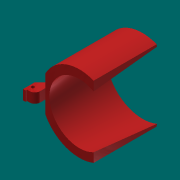
# Autodesk Inventor part: 知能ロボコン吸引部２.1.2
Saved by Autodesk Inventor 2013 (Build 170138000, 138)
## iProperties
Created: 2014-11-21
Part Number: 知能ロボコン吸引部２.1.2
Material: 一般
Document SubType Name: Modeling
Designer: horumo136
Density: 1 g/cm^3
Author: horumo136
Autodesk Inventor part; units mm, degrees
sketch "スケッチ1" plane through (0, 0, 0) normal (0, 0, 1) x (1, 0, 0)
  line L0 (0, 0) -> (32, 0)
  line L1 (0, 0) -> (0, 30)
  line L2 (0, 30) -> (35, 30)
  line L3 (35, 30) -> (32, 0)
  line L4 (32, 0) -> (33.9901, -0.199)
  line L5 (33.9901, -0.199) -> (36.9901, 29.801)
  line L6 (36.9901, 29.801) -> (35, 30)
  line L7 (0, 0) -> (0, -80)
  line L8 (0, -80) -> (26.01, -80)
  line L9 (32, 0) -> (24.0199, -79.801)
  line L10 (33.9901, -0.199) -> (26.01, -80)
  line L11 (26.01, -80) -> (24.0199, -79.801)
  line L12 (26.01, -80) -> (36.9901, -80)
  line L13 (36.9901, -80) -> (36.9901, 29.801)
  line L14 (24.0199, -79.801) -> (24, -80)
  dimension "d0" = 32
  dimension "d1" = 30
  dimension "d2" = 35
  dimension "d3" = 2
  dimension "d4" = 80
  constraints: 30 end point, 10 perpendicular, 2 parallel, 1 collinear, 1 horizontal, 1 point on line
  measures "d0" distance of L0.start L0.end
  measures "d1" distance of L0.start L1.end
  measures "d2" distance of L1.end L2.end
  measures "d3" distance of L0.end L4.end
  measures "d4" distance of L0.start L7.end
revolve "回転1" add sketch "スケッチ1" angle 360 about axis through (0, 0, 0) along (0, 1, 0) contours L3 L6 L5 L4 | L4 L10 L11 L9 | L5 L13 L12 L10 | L11 L8 L14
ref_plane "作業平面4" through (0, 0, 37) normal (0, 0, 1) x (1, 0, 0)
sketch "スケッチ2" plane through (0, 0, 37) normal (0, 0, 1) x (1, 0, 0)
  circle A0 centre (0, 0) radius 33
  line L0 (0, 0) -> (0, -46)
  line L1 (-13.5, -41) -> (13.5, -41)
  line L2 (13.5, -41) -> (13.5, -51)
  line L3 (13.5, -51) -> (-13.5, -51)
  line L4 (-13.5, -51) -> (-13.5, -41)
  line L5 (-13.5, -41) -> (13.5, -51) construction
  line L6 (13.5, -41) -> (-13.5, -51) construction
  dimension "d10" = 66
  dimension "d11" = 46
  dimension "d12" = 27
  dimension "d13" = 10
  constraints: 14 end point, 2 midpoint, 2 parallel, 1 centre point, 1 coincident, 1 horizontal, 1 perpendicular, 1 vertical
  measures "d10" diameter of A0
  measures "d11" distance of L0.start L0.end
  measures "d12" distance of L2.end L3.end
  measures "d13" distance of L1.end L2.end
sketch "スケッチ4" plane through (0, -80, 0) normal (0, -1, 0) x (1, 0, 0)
  circle A0 centre (0, 0) radius 36.9901 projected
  line L0 (-20, 25.4) -> (20, 25.4)
  line L1 (20, 25.4) -> (20, -25.4)
  line L2 (20, -25.4) -> (-20, -25.4)
  line L3 (-20, -25.4) -> (-20, 25.4)
  line L4 (-20, 25.4) -> (20, -25.4) construction
  line L5 (20, 25.4) -> (-20, -25.4) construction
  arc A1 (20, 13.2808) -> (-20, 13.2808) centre (0, 0) ccw
  arc A2 (-20, -13.2808) -> (20, -13.0826) centre (-0.0647, -0.1207) ccw
  dimension "d14" = 40
  dimension "d15" = 50.8
  constraints: 12 end point, 4 point on circle, 4 point on line, 2 centre point, 2 midpoint, 2 parallel, 1 concentric, 1 horizontal, 1 perpendicular
  measures "d14" distance of L1.end L2.end
  measures "d15" distance of L0.end L1.end
extrude "押し出し1" add sketch "スケッチ4" along normal blind 10 contours L0 L1 A1 L3 | A2 L1 L2 L3
sketch "スケッチ5" plane through (-20, -80, 25.4) normal (0, 0, 1) x (1, 0, 0)
  line L0 (0, 0) -> (40, 0) projected
  line L1 (40, 0) -> (40, -10) projected
  line L2 (20, 0) -> (20, -5)
  line L3 (20, -5) -> (35, -5)
  line L4 (20, -5) -> (5, -5)
  circle A0 centre (5, -5) radius 1.25
  circle A1 centre (35, -5) radius 1.25
  point P0 (20, 80)
  dimension "d18" = 5
  dimension "d19" = 15
  dimension "d20" = 15
  dimension "d21" = 2.5
  dimension "d22" = 2.5
  constraints: 6 end point, 2 centre point, 2 coincident, 1 collinear, 1 midpoint, 1 parallel, 1 perpendicular
  measures "d18" distance of L2.start L2.end
  measures "d19" distance of L2.end L3.end
  measures "d20" distance of L2.end L4.end
  measures "d21" diameter of A0
  measures "d22" diameter of A1
extrude "押し出し2" cut sketch "スケッチ5" against normal blind 51
extrude "押し出し3" cut sketch "スケッチ2" against normal blind 80 contours L1 L2 L3 L4
sketch "スケッチ6" plane through (0, -80, 0) normal (0, -1, 0) x (1, 0, 0)
  arc A0 (-20, -13.2808) -> (2.6513, -23.8531) centre (-0.0647, -0.1207) ccw projected
  arc A1 (20, -13.2665) -> (2.6513, -23.8531) centre (0, 0) ccw projected
  line L0 (20, -13.2665) -> (20, -25.4) projected
  line L1 (-20, -25.4) -> (-20, -13.2808) projected
  line L2 (20, 25.4) -> (20, 13.2808) projected
  arc A2 (20, 13.2808) -> (-20, 13.2808) centre (0, 0) ccw projected
  line L3 (-20, 13.2808) -> (-20, 25.4) projected
  arc A3 (-20, 13.2808) -> (-20, -13.2808) centre (0.1181, 0) ccw
  arc A4 (-20, 25.4) -> (-20, -25.4) centre (1.0675, 0) ccw
  arc A5 (20, -13.2665) -> (20, 13.2808) centre (0.0108, 0.0072) ccw
  arc A6 (20, -25.4) -> (20, 25.4) centre (-1.0675, 0) ccw
  dimension "d27" = 33
  dimension "d28" = 33
  constraints: 8 point on circle, 4 centre point, 2 tangent
  measures "d27" radius of A4
  measures "d28" radius of A6
extrude "押し出し4" add sketch "スケッチ6" along normal blind 10 contours L1 A4 L3 A3 A1 | A5 L2 A6 L0
sketch "スケッチ7" plane through (0, -51, 0) normal (0, 1, 0) x (1, 0, 0)
  arc A0 (13.5, 34.4386) -> (-13.5, 34.4386) centre (0, 0) ccw projected
  line L0 (-10, 26.9901) -> (10, 26.9901)
  line L1 (10, 26.9901) -> (10, 46.9901)
  line L2 (10, 46.9901) -> (-10, 46.9901)
  line L3 (-10, 46.9901) -> (-10, 26.9901)
  line L4 (-10, 26.9901) -> (10, 46.9901) construction
  line L5 (10, 26.9901) -> (-10, 46.9901) construction
  point P0 (0, 36.9901)
  dimension "d31" = 20
  constraints: 12 end point, 2 midpoint, 2 parallel, 1 horizontal, 1 perpendicular, 1 point on circle
  measures "d31" distance of L1.end L0.end
extrude "押し出し5" add sketch "スケッチ7" against normal blind 5
mirror "ミラー1" about plane through (0, 0, 0) normal (0, 0, 1) of "押し出し5"
ref_plane "作業平面5" through (10, -51, 41.3014) normal (0, 1, 0) x (1, 0, 0)
sketch "スケッチ8" plane through (10, -51, 41.3014) normal (0, 1, 0) x (1, 0, 0)
  line L0 (-14.9767, 1.255) -> (-4.9767, 1.255)
  line L1 (-4.9767, 1.255) -> (-4.9767, 81.255)
  line L2 (-4.9767, 81.255) -> (-14.9767, 81.255)
  line L3 (-14.9767, 81.255) -> (-14.9767, 1.255)
  line L4 (-14.9767, 1.255) -> (-4.9767, 81.255) construction
  line L5 (-4.9767, 1.255) -> (-14.9767, 81.255) construction
  line L6 (-9.9767, 81.255) -> (-9.9767, 1.255)
  circle A0 centre (-9.9767, 81.255) radius 1
  circle A1 centre (-9.9767, 1.255) radius 1
  point P0 (-9.9767, 41.255)
  dimension "d42" = 10
  dimension "d43" = 80
  dimension "d44" = 2
  dimension "d45" = 2
  constraints: 14 end point, 4 midpoint, 2 centre point, 2 coincident, 2 parallel, 1 horizontal, 1 perpendicular
  measures "d42" distance of L2.end L1.end
  measures "d43" distance of L1.end L0.end
  measures "d44" diameter of A0
  measures "d45" diameter of A1
extrude "押し出し7" cut sketch "スケッチ8" against normal blind 5 contours L6 A1 L0 | L0 A1 | L0 A1 L6 | A0 L2 L6 | L6 L2 A0 | L2 A0
ref_plane "作業平面6" through (-10, -53.5, -46.9901) normal (0, 0, -1) x (-1, 0, 0)
sketch "スケッチ9" plane through (-10, -53.5, -46.9901) normal (0, 0, -1) x (-1, 0, 0)
  line L0 (26.829, -26.5556) -> (-47.1085, -26.5556)
  line L1 (-0.028, -26.5556) -> (-0.028, 22.4444)
  line L2 (-23.7626, 22.4444) -> (28.9336, 22.4444)
  line L3 (28.9336, 22.4444) -> (28.9336, 86.0653)
  line L4 (28.9336, 86.0653) -> (-23.7626, 86.0653)
  line L5 (-23.7626, 86.0653) -> (-23.7626, 22.4444)
  line L6 (-23.7626, 86.0653) -> (-48.5643, 86.0653)
  line L7 (-48.5643, 86.0653) -> (-48.5643, -39.6917)
  line L8 (-48.5643, -39.6917) -> (-23.7626, -39.6917)
  line L9 (-23.7626, -39.6917) -> (-23.7626, 86.0653)
  line L10 (-23.7626, 22.4444) -> (28.9336, 22.4444)
  line L11 (28.9336, 22.4444) -> (28.9336, -39.6917)
  line L12 (28.9336, -39.6917) -> (-23.7626, -39.6917)
  line L13 (-23.7626, -39.6917) -> (-23.7626, 22.4444)
  point P0 (-10, 53.5)
  dimension "d48" = 49
  constraints: 28 end point, 6 parallel, 4 horizontal, 4 perpendicular, 1 point on line
  measures "d48" distance of L1.start L1.end
extrude "押し出し9" cut sketch "スケッチ9" against normal blind 95 contours L1 L2 L11 L12 L9 L0 | L0 L9 L2 L1 | L9 L8 L7 L6 L5
sketch "スケッチ10" plane through (0, -31.0556, 0) normal (0, -1, 0) x (1, 0, 0)
  arc A0 (13.7626, 34.3345) -> (13.7626, -34.3345) centre (0, 0) ccw projected
  arc A1 (13.7626, 25.4063) -> (13.7626, -25.4063) centre (0, 0) ccw projected
  line L0 (13.7626, 25.4063) -> (13.7626, 34.3345) projected
  line L1 (-28.8944, 0) -> (-32.8944, 0)
  line L2 (-32.8944, 0) -> (-32.8944, 16.9181)
  line L3 (-32.8944, 0) -> (-32.8944, -16.9181)
  dimension "d53" = 4
  constraints: 6 end point, 3 point on circle, 2 perpendicular, 1 collinear
  measures "d53" distance of L1.start L1.end
extrude "押し出し10" cut sketch "スケッチ10" against normal blind 30 contours L2 L3 A0
sketch "スケッチ11" plane through (-32.8944, -31.0556, -16.9181) normal (-1, 0, 0) x (0, 0, 1)
  line L0 (33.8361, 0) -> (0, 0) projected
  line L1 (0, 0) -> (0, 30) projected
  line L2 (16.9181, 0) -> (16.9181, 5)
  line L3 (12.1681, 10) -> (21.6681, 10)
  line L4 (21.6681, 10) -> (21.6681, 0)
  line L5 (21.6681, 0) -> (12.1681, 0)
  line L6 (12.1681, 0) -> (12.1681, 10)
  line L7 (12.1681, 10) -> (21.6681, 0) construction
  line L8 (21.6681, 10) -> (12.1681, 0) construction
  point P0 (16.9181, 31.0556)
  dimension "d56" = 5
  dimension "d57" = 9.5
  constraints: 14 end point, 3 midpoint, 3 parallel, 1 horizontal, 1 perpendicular, 1 point on line
  measures "d56" distance of L2.start L2.end
  measures "d57" distance of L4.end L5.end
extrude "押し出し11" add sketch "スケッチ11" along normal blind 10
sketch "スケッチ12" plane through (0, -31.0556, 0) normal (0, -1, 0) x (1, 0, 0)
  line L0 (-42.8944, 4.75) -> (-32.8944, 4.75)
  line L1 (-32.8944, 4.75) -> (-32.8944, -4.75)
  line L2 (-32.8944, -4.75) -> (-42.8944, -4.75)
  line L3 (-42.8944, -4.75) -> (-42.8944, 4.75)
  line L4 (-42.8944, 4.75) -> (-32.8944, -4.75) construction
  line L5 (-32.8944, 4.75) -> (-42.8944, -4.75) construction
  point P0 (-37.8944, 0)
  constraints: 12 end point, 2 midpoint, 2 parallel, 1 horizontal, 1 perpendicular
extrude "押し出し12" add sketch "スケッチ12" along normal blind 10
sketch "スケッチ13" plane through (-42.8944, -21.0556, 4.75) normal (0, 0, 1) x (1, 0, 0)
  line L0 (0, 0) -> (0, -20) projected
  line L1 (0, -20) -> (0, -15)
  line L2 (0, -15) -> (3, -15)
  circle A0 centre (3, -15) radius 1.5
  point P0 (42.8944, 21.0556)
  dimension "d62" = 3
  dimension "d63" = 3
  constraints: 4 end point, 1 centre point, 1 coincident, 1 perpendicular, 1 point on line
  measures "d62" distance of L1.end L2.end
  measures "d63" diameter of A0
extrude "押し出し13" cut sketch "スケッチ13" against normal blind 10
chamfer "面取り1" distance 10 angle 45 1 edges at (-42.8944, -21.0556, 0)
fillet "フィレット2" radius 5 1 edges at (-32.8944, -41.0556, 0)
sketch "スケッチ14" plane through (0, -41.0556, 0) normal (0, -1, 0) x (1, 0, 0)
  line L0 (-42.8944, -4.75) -> (-37.8944, -4.75) projected
  line L1 (-42.8944, 4.75) -> (-40.3944, 4.75)
  line L2 (-40.3944, 4.75) -> (-40.3944, -4.75)
  line L3 (-40.3944, -4.75) -> (-42.8944, -4.75)
  line L4 (-42.8944, -4.75) -> (-42.8944, 4.75)
  point P0 (0, 0)
  constraints: 8 end point, 2 parallel, 1 horizontal, 1 midpoint, 1 perpendicular
extrude "押し出し14" add sketch "スケッチ14" along normal blind 1.4
